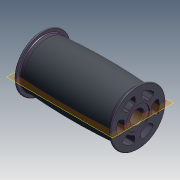
# Autodesk Inventor part: J005553
Saved by Autodesk Inventor 2015 SP1 (Build 190203100, 203)
## iProperties
Created: 2014-11-17
Material: VERO BLACK
Document SubType Name: Modeling
Designer: ARNOLDJ
Mass: 16.6292 g
Surface Area: 162.186 cm^2
Volume: 14.213 cm^3
Density: 1.17 g/cm^3
Description: NRB DRIVE ROLLER
Project: COMMON
Vendor: HHMI: JRC - ID&F
Appearance: Black Anodize
Part Number: J005553
Translation Standard: STEP AP203
FileName: 26593
PreProcessor: PRO/ENGINEER BY PARAMETRIC TECHNOLOGY CORPORATION, 2005030
PostProcessor: Build: 219, Release: 2012 SP2 - Date: Fri 04/27/2012
Sent Units: millimeter
Uncertainty: 0.0032371533199349995
ALTERED ITEM DESCRIPTION: N/A
ALTERED ITEM PART NUMBER: N/A
ALTERED ITEM VENDOR: N/A
DESIGN DEPARTMENT: HHMI: JRC - ID&F
LAB/DEPT: COMMON
REQUESTING SCIENTIST: COMMON
SPECIAL FINISH: NONE
SURFACE ROUGHNESS: N/A
Revision Number: -
Autodesk Inventor part; units mm, degrees
ref_plane "YZ Plane" through (0, 0, 0) normal (1, 0, 0) x (0, 1, 0)
ref_plane "XY Plane" through (0, 0, 0) normal (0, 0, 1) x (1, 0, 0)
sketch "Sketch10" plane through (0, 0, 0) normal (0, 0, 1) x (1, 0, 0)
  line L0 (-33.9598, 0) -> (33.9598, 0) projected
  line L1 (24.257, -12.7) -> (-24.257, -12.7) construction
  line L2 (-24.257, -12.7) -> (-24.257, 12.7) construction
  line L3 (-24.257, 12.7) -> (24.257, 12.7) construction
  line L4 (24.257, 12.7) -> (24.257, -12.7) construction
  line L5 (24.257, -12.7) -> (-24.257, 12.7) construction
  line L6 (-24.257, -12.7) -> (24.257, 12.7) construction
  line L7 (-24.257, 13.97) -> (-23.495, 13.97)
  line L8 (-23.495, 13.97) -> (-23.495, 11.938)
  line L9 (24.257, 13.97) -> (23.495, 13.97)
  line L10 (23.495, 13.97) -> (23.495, 11.938)
  line L11 (-24.257, 13.97) -> (-24.257, 0)
  line L12 (24.257, 13.97) -> (24.257, 0)
  line L13 (-24.257, 0) -> (24.257, 0)
  arc A0 (21.59, 11.938) -> (-21.59, 11.938) centre (0, -293.5393) ccw
  line L14 (-23.495, 11.938) -> (-21.59, 11.938)
  line L15 (21.59, 11.938) -> (23.495, 11.938)
  point P0 (0, 0)
  dimension "d72" = 48.514
  dimension "d73" = 25.4
  dimension "d74" = 0.762
  dimension "d75" = 1.27
  dimension "d80" = 1.905
  dimension "d81" = 0.762
  dimension "d82" = 46.99
  constraints: 30 end point, 7 perpendicular, 3 collinear, 3 horizontal, 3 midpoint, 2 horizontal alignment, 2 parallel, 2 point on circle, 2 vertical alignment, 1 centre point, 1 point on line, 1 tangent
  measures "d72" distance of L2.end L3.end
  measures "d73" distance of L1.end L2.end
  measures "d74" distance of L7.start L7.end
  measures "d75" distance between parallel lines of L7 L3
  measures "d80" distance of L8.end L14.end
  measures "d81" distance between parallel lines of L3 L14
  measures "d82" distance between parallel lines of L10 L8
revolve "Revolution3" add sketch "Sketch10" angle 360 about axis through (0, 0, 0) along (1, 0, 0)
sketch "Sketch11" plane through (0, 0, 0) normal (1, 0, 0) x (0, 1, 0)
  circle A0 centre (0, 0) radius 1.5875
  dimension "d84" = 3.175
  constraints: 2 coincident, 1 centre point
  measures "d84" diameter of A0
extrude "Extrusion5" cut sketch "Sketch11" along normal up to surface (48.514 mm away) from surface at -24.257
fillet "Fillet5" radius 0.381 6 edges at (-23.495, -11.938, 0) (23.495, -11.938, 0) (23.495, -13.97, 0) (24.257, -13.97, 0) (-24.257, -13.97, 0) (-23.495, -13.97, 0)
hole "Hole5" at (-24.257, 0, 0) direction (1, 0, 0) diameter 6.3246 end through all counterbore diameter 11.684 counterbore depth 0.508
hole "Hole6" at (24.257, 0, 0) direction (-1, 0, 0) diameter 4.7752 end through all counterbore diameter 11.684 counterbore depth 0.508
sketch "Sketch12" plane through (0, 0, 0) normal (1, 0, 0) x (0, 1, 0)
  circle A0 centre (0, 0) radius 11.938 projected
  circle A1 centre (0, 0) radius 5.842 projected
  line L0 (0, 21.1582) -> (0, -21.1582) projected
  line L1 (-21.1582, 0) -> (21.1582, 0) projected
  circle A2 centre (0, 0) radius 5.842 projected
  line L2 (-2.0816, 6.6676) -> (-3.7012, 10.1407)
  line L3 (2.401, 6.5594) -> (4.015, 10.0206)
  arc A3 (2.401, 6.5594) -> (-2.0816, 6.6676) centre (0, 0) ccw
  arc A4 (4.015, 10.0206) -> (-3.7012, 10.1407) centre (0, 0) ccw
  dimension "d112" = 25
  dimension "d113" = 25
  dimension "d114" = 10.795
  dimension "d115" = 6.985
  constraints: 6 point on circle, 4 end point, 2 centre point, 2 coincident
  measures "d112" angle of L0 L2
  measures "d113" angle of L0 L3
  measures "d114" radius of A4
  measures "d115" radius of A3
extrude "Extrusion6" cut sketch "Sketch12" along normal mid plane 73.66 contours A4 L3 A3 L0 | L0 A3 L2 A4
fillet "Fillet6" radius 1.016 4 edges at (0, 4.015, 10.0206) (0, 2.401, 6.5594) (0, -2.0816, 6.6676) (0, -3.7012, 10.1407)
pattern_circular "Circular Pattern1" count 6 over 360 about axis through (-10, 0, 0) along (1, 0, 0) of "Extrusion6", "Fillet6"
sketch "Sketch13" plane through (0, 0, 0) normal (1, 0, 0) x (0, 1, 0)
  line L0 (0, 15.113) -> (0, -15.113) projected
  line L1 (-15.113, 0) -> (15.113, 0) projected
  circle A0 centre (0, 0) radius 10.795
  dimension "d122" = 21.59
  constraints: 1 centre point, 1 coincident
  measures "d122" diameter of A0
extrude "Extrusion7" cut sketch "Sketch13" along normal mid plane 36.83
chamfer "Chamfer3" distance 0.508 angle 45 2 edges at (23.749, 0, -3.1623) (-23.749, 0, -3.1623)
